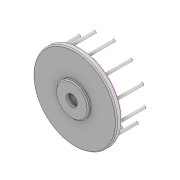
# Autodesk Inventor part: base
Saved by Autodesk Inventor 2021 (Build 250183000, 183)
## iProperties
Created: 2021-06-23
Part Number: base
Material: Generic
Document SubType Name: Modeling
Designer: Hp
Density: 1 g/cm^3
Appearance: Default
Author: Hp
Autodesk Inventor part; units mm, degrees
ref_plane "YZ Plane" through (0, 0, 0) normal (1, 0, 0) x (0, 1, 0)
ref_plane "XZ Plane" through (0, 0, 0) normal (0, 1, 0) x (-1, 0, 0)
ref_plane "XY Plane" through (0, 0, 0) normal (0, 0, 1) x (1, 0, 0)
sketch "Sketch1" plane through (0, 0, 0) normal (0, 0, 1) x (1, 0, 0)
  point P0 (0, 0)
sketch "Sketch2" plane through (0, 0, 0) normal (0, 0, 1) x (1, 0, 0)
  circle A0 centre (0, 0) radius 75
  line L0 (-65.0875, -9.525) -> (-104.775, -39.6875) construction
  line L1 (-104.775, -39.6875) -> (-119.0625, -20.6375) construction
  line L2 (-119.0625, -20.6375) -> (-158.75, -15.875) construction
  line L3 (-158.75, -15.875) -> (-179.3875, -52.3875) construction
  spline S0 degree 4 poles (-65.0875, -9.525) (-104.775, -39.6875) (-119.0625, -20.6375) (-158.75, -15.875) (-179.3875, -52.3875) knots 1 1 1 1 1 2 2 2 2 2
  circle A1 centre (-65.0875, -9.525) radius 2.5
  dimension "d0" = 150
  dimension "d87" = 5
  constraints: 2 centre point, 2 coincident, 3 other
  measures "d0" diameter of A0
  measures "d87" diameter of A1
extrude "Extrusion1" add sketch "Sketch2" along normal blind 10 contours A0 | A1
hole "Hole1" at (0, 0, 0) direction (0, 0, 1) diameter 5 end through all
sketch "Sketch3" plane through (0, 0, 10) normal (0, 0, 1) x (1, 0, 0)
  point P0 (0, 0)
sketch "Sketch4" plane through (0, 0, 10) normal (0, 0, 1) x (1, 0, 0)
  point P0 (0, 0)
hole "Hole2" at (0, 0, 10) direction (0, 0, -1) diameter 20 end through all
chamfer "Chamfer1" distance 2 angle 45 1 edges at (0, 10, 10)
fillet "Fillet1" radius 2 1 edges at (-75, 0, 10)
fillet "Fillet2" radius 2 1 edges at (-75, 0, 0)
sketch "Sketch8" plane through (0, 0, 10) normal (0, 0, 1) x (1, 0, 0)
  circle A0 centre (0, 0) radius 10 projected
  circle A1 centre (0, 0) radius 29.2721
  constraints: 1 centre point, 1 coincident
extrude "Extrusion4" add sketch "Sketch8" along normal blind 5
chamfer "Chamfer2" distance 2 angle 45 1 edges at (-29.2721, 0, 15)
sketch "Sketch24" plane through (0, 0, 0) normal (1, 0, 0) x (0, 1, 0)
  line L0 (10, 0) -> (-10, 0) projected
  point P0 (0, 0)
sketch "Sketch25" plane through (0, 0, 0) normal (0, 0, 1) x (1, 0, 0)
  circle A0 centre (0, 0) radius 10 projected
  circle A1 centre (0, 0) radius 73 projected
  circle A2 centre (23.8125, -61.9125) radius 2.5
  circle A3 centre (51.5785, -41.7115) radius 2.5
  circle A4 centre (65.524, -10.334) radius 2.5
  circle A5 centre (61.9125, 23.8125) radius 2.5
  circle A6 centre (41.7115, 51.5785) radius 2.5
  circle A7 centre (10.334, 65.524) radius 2.5
  circle A8 centre (-23.8125, 61.9125) radius 2.5
  circle A9 centre (-51.5785, 41.7115) radius 2.5
  circle A10 centre (-65.524, 10.334) radius 2.5
  circle A11 centre (-61.9125, -23.8125) radius 2.5
  circle A12 centre (-41.7115, -51.5785) radius 2.5
  circle A13 centre (-10.334, -65.524) radius 2.5
  circle A14 centre (0, 0) radius 10 projected
  circle A15 centre (0, 0) radius 10 projected
  dimension "d104" = 5
  dimension "d107" = 360
  constraints: 12 centre point, 2 coincident, 25 other
  measures "d104" diameter of A2
sketch "Sketch26" plane through (0, 0, 0) normal (0, 0, -1) x (-1, 0, 0)
  point P0 (0, 0)
extrude "Extrusion6" add sketch "Sketch25" against normal blind 50 contours A3 | A4 | A5 | A6 | A7 | A8 | A9 | A10 | A11 | A12 | A13
sketch "Sketch28" plane through (0, 0, 0) normal (0, 0, -1) x (-1, 0, 0)
  circle A0 centre (-51.5785, -41.7115) radius 2.5 projected
  circle A1 centre (65.524, 10.334) radius 2.5 projected
  circle A2 centre (-51.5785, -41.7115) radius 2.5 projected
  circle A3 centre (-10.334, 65.524) radius 2.5 projected
  circle A4 centre (-65.524, -10.334) radius 2.5 projected
  circle A5 centre (61.9125, -23.8125) radius 2.5 projected
  circle A6 centre (51.5785, 41.7115) radius 2.5 projected
  circle A7 centre (10.334, -65.524) radius 2.5 projected
  circle A8 centre (-41.7115, 51.5785) radius 2.5 projected
  circle A9 centre (-61.9125, 23.8125) radius 2.5 projected
  circle A10 centre (41.7115, -51.5785) radius 2.5 projected
  circle A11 centre (23.8125, 61.9125) radius 2.5 projected
  circle A12 centre (0, 0) radius 10 projected
  circle A13 centre (0, 0) radius 73 projected
  circle A14 centre (65.524, 10.334) radius 2.5 projected
  circle A15 centre (-51.5785, -41.7115) radius 2.5 projected
  circle A16 centre (-10.334, 65.524) radius 2.5 projected
  circle A17 centre (-65.524, -10.334) radius 2.5 projected
  circle A18 centre (61.9125, -23.8125) radius 2.5 projected
  circle A19 centre (51.5785, 41.7115) radius 2.5 projected
  circle A20 centre (10.334, -65.524) radius 2.5 projected
  circle A21 centre (-41.7115, 51.5785) radius 2.5 projected
  circle A22 centre (-61.9125, 23.8125) radius 2.5 projected
  circle A23 centre (41.7115, -51.5785) radius 2.5 projected
  circle A24 centre (23.8125, 61.9125) radius 2.5 projected
  circle A25 centre (0, 0) radius 10 projected
  circle A26 centre (0, 0) radius 73 projected
  circle A27 centre (65.524, 10.334) radius 2.5 projected
  circle A28 centre (-51.5785, -41.7115) radius 2.5 projected
  circle A29 centre (-10.334, 65.524) radius 2.5 projected
  circle A30 centre (-65.524, -10.334) radius 2.5 projected
  circle A31 centre (61.9125, -23.8125) radius 2.5 projected
  circle A32 centre (51.5785, 41.7115) radius 2.5 projected
  circle A33 centre (10.334, -65.524) radius 2.5 projected
  circle A34 centre (-41.7115, 51.5785) radius 2.5 projected
  circle A35 centre (-61.9125, 23.8125) radius 2.5 projected
  circle A36 centre (41.7115, -51.5785) radius 2.5 projected
  circle A37 centre (23.8125, 61.9125) radius 2.5 projected
  circle A38 centre (0, 0) radius 10 projected
  circle A39 centre (0, 0) radius 73 projected
sketch "Sketch29" plane through (0, 0, 0) normal (0, 0, 1) x (1, 0, 0)
  circle A0 centre (23.8125, -61.9125) radius 2.5
  point P0 (0, 0)
  dimension "d111" = 5
  constraints: 1 centre point
  measures "d111" diameter of A0
extrude "Extrusion7" add sketch "Sketch29" against normal blind 50
body "Solid1"
